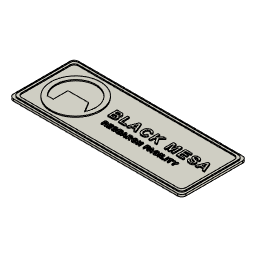
black_mesa_patch (Autodesk Fusion 360 design; units mm, degrees)
Autodesk Fusion 360 part; units mm, degrees
sketch "Sketch1" plane through (0, 0, 0) normal (0, 0, 1) x (1, 0, 0)
  line L0 (155.8764, -60.5348) -> (155.8764, -66.4765)
  line L1 (155.8764, -66.4765) -> (160.0294, -66.4765)
  spline S0 degree 3 poles (160.0294, -66.4765) (161.646, -66.4765) (162.6717, -66.4315) (163.1065, -66.3407) knots 0 0 0 0 1 1 1 1
  spline S1 degree 3 poles (163.1065, -66.3407) (163.7733, -66.219) (164.3166, -65.9235) (164.7355, -65.4534) knots 0 0 0 0 1 1 1 1
  spline S2 degree 3 poles (164.7355, -65.4534) (165.1553, -64.9833) (165.3643, -64.3545) (165.3643, -63.5661) knots 0 0 0 0 1 1 1 1
  spline S3 degree 3 poles (165.3643, -63.5661) (165.3643, -62.8993) (165.2029, -62.334) (164.8792, -61.8683) knots 0 0 0 0 1 1 1 1
  spline S4 degree 3 poles (164.8792, -61.8683) (164.5565, -61.4035) (164.089, -61.0657) (163.4778, -60.8532) knots 0 0 0 0 1 1 1 1
  spline S5 degree 3 poles (163.4778, -60.8532) (162.8658, -60.6407) (161.5402, -60.5348) (159.4985, -60.5348) knots 0 0 0 0 1 1 1 1
  line L2 (159.4985, -60.5348) -> (155.8764, -60.5348)
  line L3 (155.8764, -51.6977) -> (155.8764, -56.8368)
  line L4 (155.8764, -56.8368) -> (158.8168, -56.8368)
  spline S6 degree 3 poles (158.8168, -56.8368) (160.5648, -56.8368) (161.6513, -56.8112) (162.0755, -56.761) knots 0 0 0 0 1 1 1 1
  spline S7 degree 3 poles (162.0755, -56.761) (162.8437, -56.6701) (163.447, -56.4047) (163.8871, -55.9646) knots 0 0 0 0 1 1 1 1
  spline S8 degree 3 poles (163.8871, -55.9646) (164.3263, -55.5254) (164.5468, -54.9468) (164.5468, -54.2298) knots 0 0 0 0 1 1 1 1
  spline S9 degree 3 poles (164.5468, -54.2298) (164.5468, -53.5419) (164.3571, -52.9836) (163.9779, -52.555) knots 0 0 0 0 1 1 1 1
  spline S10 degree 3 poles (163.9779, -52.555) (163.5987, -52.1255) (163.036, -51.8644) (162.2881, -51.7736) knots 0 0 0 0 1 1 1 1
  spline S11 degree 3 poles (162.2881, -51.7736) (161.8436, -51.7233) (160.5648, -51.6977) (158.4534, -51.6977) knots 0 0 0 0 1 1 1 1
  line L5 (158.4534, -51.6977) -> (155.8764, -51.6977)
  line L6 (151.3899, -47.9997) -> (160.272, -47.9997)
  spline S12 degree 3 poles (160.272, -47.9997) (162.0306, -47.9997) (163.3411, -48.0729) (164.2054, -48.2193) knots 0 0 0 0 1 1 1 1
  spline S13 degree 3 poles (164.2054, -48.2193) (165.0689, -48.3666) (165.8423, -48.6718) (166.5241, -49.1366) knots 0 0 0 0 1 1 1 1
  spline S14 degree 3 poles (166.5241, -49.1366) (167.2067, -49.6014) (167.7747, -50.2205) (168.2298, -50.9931) knots 0 0 0 0 1 1 1 1
  spline S15 degree 3 poles (168.2298, -50.9931) (168.684, -51.7665) (168.9115, -52.6335) (168.9115, -53.593) knots 0 0 0 0 1 1 1 1
  spline S16 degree 3 poles (168.9115, -53.593) (168.9115, -54.6337) (168.631, -55.5889) (168.0701, -56.4576) knots 0 0 0 0 1 1 1 1
  spline S17 degree 3 poles (168.0701, -56.4576) (167.5092, -57.3263) (166.749, -57.9789) (165.7894, -58.4129) knots 0 0 0 0 1 1 1 1
  spline S18 degree 3 poles (165.7894, -58.4129) (167.1432, -58.8071) (168.1839, -59.4791) (168.9115, -60.429) knots 0 0 0 0 1 1 1 1
  spline S19 degree 3 poles (168.9115, -60.429) (169.6391, -61.3788) (170.0033, -62.4954) (170.0033, -63.7786) knots 0 0 0 0 1 1 1 1
  spline S20 degree 3 poles (170.0033, -63.7786) (170.0033, -64.7893) (169.7679, -65.7718) (169.2978, -66.727) knots 0 0 0 0 1 1 1 1
  spline S21 degree 3 poles (169.2978, -66.727) (168.8286, -67.6812) (168.1865, -68.4441) (167.3734, -69.0156) knots 0 0 0 0 1 1 1 1
  spline S22 degree 3 poles (167.3734, -69.0156) (166.5593, -69.5862) (165.5566, -69.9381) (164.3642, -70.0686) knots 0 0 0 0 1 1 1 1
  spline S23 degree 3 poles (164.3642, -70.0686) (163.6163, -70.1498) (161.8127, -70.2) (158.9535, -70.2203) knots 0 0 0 0 1 1 1 1
  line L7 (158.9535, -70.2203) -> (151.3899, -70.2203)
  line L8 (151.3899, -70.2203) -> (151.3899, -47.9997)
  line L9 (177.1731, -70.2203) -> (177.1731, -48.1814)
  line L10 (177.1731, -48.1814) -> (181.6596, -48.1814)
  line L11 (181.6596, -48.1814) -> (181.6596, -66.4765)
  line L12 (181.6596, -66.4765) -> (192.8153, -66.4765)
  line L13 (192.8153, -66.4765) -> (192.8153, -70.2203)
  line L14 (192.8153, -70.2203) -> (177.1731, -70.2203)
  line L15 (211.0496, -61.4293) -> (207.9875, -53.1831)
  line L16 (207.9875, -53.1831) -> (204.9871, -61.4293)
  line L17 (204.9871, -61.4293) -> (211.0496, -61.4293)
  line L18 (219.3107, -70.2205) -> (214.4301, -70.2205)
  line L19 (214.4301, -70.2205) -> (212.4898, -65.1731)
  line L20 (212.4898, -65.1731) -> (203.6077, -65.1731)
  line L21 (203.6077, -65.1731) -> (201.7733, -70.2205)
  line L22 (201.7733, -70.2205) -> (197.0143, -70.2205)
  line L23 (197.0143, -70.2205) -> (205.6688, -47.9999)
  line L24 (205.6688, -47.9999) -> (210.4128, -47.9999)
  line L25 (210.4128, -47.9999) -> (219.3107, -70.2205)
  line L26 (239.1675, -62.0507) -> (243.5182, -63.4301)
  spline S24 degree 3 poles (243.5182, -63.4301) (242.8505, -65.8545) (241.7411, -67.6563) (240.1906, -68.8329) knots 0 0 0 0 1 1 1 1
  spline S25 degree 3 poles (240.1906, -68.8329) (238.6384, -70.0111) (236.6716, -70.5994) (234.2869, -70.5994) knots 0 0 0 0 1 1 1 1
  spline S26 degree 3 poles (234.2869, -70.5994) (231.3359, -70.5994) (228.9105, -69.5913) (227.0117, -67.5752) knots 0 0 0 0 1 1 1 1
  spline S27 degree 3 poles (227.0117, -67.5752) (225.1111, -65.56) (224.1613, -62.8039) (224.1613, -59.307) knots 0 0 0 0 1 1 1 1
  spline S28 degree 3 poles (224.1613, -59.307) (224.1613, -55.609) (225.1164, -52.7365) (227.0258, -50.6904) knots 0 0 0 0 1 1 1 1
  spline S29 degree 3 poles (227.0258, -50.6904) (228.9361, -48.6443) (231.447, -47.6212) (234.5594, -47.6212) knots 0 0 0 0 1 1 1 1
  spline S30 degree 3 poles (234.5594, -47.6212) (237.2775, -47.6212) (239.485, -48.4238) (241.1828, -50.0307) knots 0 0 0 0 1 1 1 1
  spline S31 degree 3 poles (241.1828, -50.0307) (242.1935, -50.9805) (242.9511, -52.3449) (243.4564, -54.1238) knots 0 0 0 0 1 1 1 1
  line L27 (243.4564, -54.1238) -> (239.0158, -55.1839)
  spline S32 degree 3 poles (239.0158, -55.1839) (238.7521, -54.0321) (238.2045, -53.1228) (237.371, -52.456) knots 0 0 0 0 1 1 1 1
  spline S33 degree 3 poles (237.371, -52.456) (236.5376, -51.7893) (235.5242, -51.4559) (234.3327, -51.4559) knots 0 0 0 0 1 1 1 1
  spline S34 degree 3 poles (234.3327, -51.4559) (232.6844, -51.4559) (231.3491, -52.0468) (230.3234, -53.2295) knots 0 0 0 0 1 1 1 1
  spline S35 degree 3 poles (230.3234, -53.2295) (229.2977, -54.4113) (228.7853, -56.326) (228.7853, -58.9736) knots 0 0 0 0 1 1 1 1
  spline S36 degree 3 poles (228.7853, -58.9736) (228.7853, -61.7826) (229.2898, -63.7837) (230.3005, -64.9761) knots 0 0 0 0 1 1 1 1
  spline S37 degree 3 poles (230.3005, -64.9761) (231.3112, -66.1685) (232.6244, -66.7647) (234.241, -66.7647) knots 0 0 0 0 1 1 1 1
  spline S38 degree 3 poles (234.241, -66.7647) (235.4334, -66.7647) (236.4591, -66.3855) (237.3181, -65.6279) knots 0 0 0 0 1 1 1 1
  spline S39 degree 3 poles (237.3181, -65.6279) (238.1771, -64.8694) (238.7936, -63.6779) (239.1675, -62.0507) knots 0 0 0 0 1 1 1 1
  line L28 (250.6879, -70.2203) -> (250.6879, -47.9997)
  line L29 (250.6879, -47.9997) -> (255.1744, -47.9997)
  line L30 (255.1744, -47.9997) -> (255.1744, -57.8669)
  line L31 (255.1744, -57.8669) -> (264.2381, -47.9997)
  line L32 (264.2381, -47.9997) -> (270.2706, -47.9997)
  line L33 (270.2706, -47.9997) -> (261.9045, -56.6543)
  line L34 (261.9045, -56.6543) -> (270.7257, -70.2203)
  line L35 (270.7257, -70.2203) -> (264.9208, -70.2203)
  line L36 (264.9208, -70.2203) -> (258.8115, -59.7922)
  line L37 (258.8115, -59.7922) -> (255.1744, -63.5061)
  line L38 (255.1744, -63.5061) -> (255.1744, -70.2203)
  line L39 (255.1744, -70.2203) -> (250.6879, -70.2203)
  line L40 (288.1267, -70.2203) -> (288.1267, -47.9997)
  line L41 (288.1267, -47.9997) -> (294.8409, -47.9997)
  line L42 (294.8409, -47.9997) -> (298.8731, -63.1568)
  line L43 (298.8731, -63.1568) -> (302.8595, -47.9997)
  line L44 (302.8595, -47.9997) -> (309.5888, -47.9997)
  line L45 (309.5888, -47.9997) -> (309.5888, -70.2203)
  line L46 (309.5888, -70.2203) -> (305.4207, -70.2203)
  line L47 (305.4207, -70.2203) -> (305.4207, -52.7287)
  line L48 (305.4207, -52.7287) -> (301.0101, -70.2203)
  line L49 (301.0101, -70.2203) -> (296.6903, -70.2203)
  line L50 (296.6903, -70.2203) -> (292.2947, -52.7287)
  line L51 (292.2947, -52.7287) -> (292.2947, -70.2203)
  line L52 (292.2947, -70.2203) -> (288.1267, -70.2203)
  line L53 (317.3049, -70.2203) -> (317.3049, -47.9997)
  line L54 (317.3049, -47.9997) -> (333.7814, -47.9997)
  line L55 (333.7814, -47.9997) -> (333.7814, -51.7586)
  line L56 (333.7814, -51.7586) -> (321.7914, -51.7586)
  line L57 (321.7914, -51.7586) -> (321.7914, -56.6851)
  line L58 (321.7914, -56.6851) -> (332.9471, -56.6851)
  line L59 (332.9471, -56.6851) -> (332.9471, -60.429)
  line L60 (332.9471, -60.429) -> (321.7914, -60.429)
  line L61 (321.7914, -60.429) -> (321.7914, -66.4765)
  line L62 (321.7914, -66.4765) -> (334.2056, -66.4765)
  line L63 (334.2056, -66.4765) -> (334.2056, -70.2203)
  line L64 (334.2056, -70.2203) -> (317.3049, -70.2203)
  line L65 (340.1321, -62.9903) -> (344.4977, -62.5661)
  spline S40 degree 3 poles (344.4977, -62.5661) (344.7605, -64.031) (345.2941, -65.107) (346.0967, -65.794) knots 0 0 0 0 1 1 1 1
  spline S41 degree 3 poles (346.0967, -65.794) (346.9001, -66.4811) (347.9832, -66.825) (349.3475, -66.825) knots 0 0 0 0 1 1 1 1
  spline S42 degree 3 poles (349.3475, -66.825) (350.793, -66.825) (351.8814, -66.519) (352.6143, -65.9078) knots 0 0 0 0 1 1 1 1
  spline S43 degree 3 poles (352.6143, -65.9078) (353.3463, -65.2966) (353.7132, -64.5822) (353.7132, -63.7629) knots 0 0 0 0 1 1 1 1
  spline S44 degree 3 poles (353.7132, -63.7629) (353.7132, -63.2382) (353.5597, -62.791) (353.251, -62.4215) knots 0 0 0 0 1 1 1 1
  spline S45 degree 3 poles (353.251, -62.4215) (352.9423, -62.0528) (352.4044, -61.7327) (351.6371, -61.4593) knots 0 0 0 0 1 1 1 1
  spline S46 degree 3 poles (351.6371, -61.4593) (351.1105, -61.2776) (349.9137, -60.9539) (348.0449, -60.4891) knots 0 0 0 0 1 1 1 1
  spline S47 degree 3 poles (348.0449, -60.4891) (345.639, -59.8929) (343.9518, -59.1609) (342.9817, -58.2913) knots 0 0 0 0 1 1 1 1
  spline S48 degree 3 poles (342.9817, -58.2913) (341.6182, -57.069) (340.9355, -55.5785) (340.9355, -53.8208) knots 0 0 0 0 1 1 1 1
  spline S49 degree 3 poles (340.9355, -53.8208) (340.9355, -52.6883) (341.2557, -51.63) (341.8986, -50.6449) knots 0 0 0 0 1 1 1 1
  spline S50 degree 3 poles (341.8986, -50.6449) (342.5389, -49.6597) (343.4641, -48.9092) (344.6715, -48.3941) knots 0 0 0 0 1 1 1 1
  spline S51 degree 3 poles (344.6715, -48.3941) (345.8797, -47.8782) (347.3367, -47.6207) (349.0441, -47.6207) knots 0 0 0 0 1 1 1 1
  spline S52 degree 3 poles (349.0441, -47.6207) (351.8337, -47.6207) (353.9328, -48.2328) (355.343, -49.4551) knots 0 0 0 0 1 1 1 1
  spline S53 degree 3 poles (355.343, -49.4551) (356.7523, -50.6775) (357.4923, -52.31) (357.5637, -54.3508) knots 0 0 0 0 1 1 1 1
  line L66 (357.5637, -54.3508) -> (353.0773, -54.5475)
  spline S54 degree 3 poles (353.0773, -54.5475) (352.885, -53.4062) (352.4723, -52.5851) (351.8408, -52.0842) knots 0 0 0 0 1 1 1 1
  spline S55 degree 3 poles (351.8408, -52.0842) (351.2102, -51.5841) (350.2621, -51.3346) (348.9992, -51.3346) knots 0 0 0 0 1 1 1 1
  spline S56 degree 3 poles (348.9992, -51.3346) (347.6957, -51.3346) (346.6752, -51.6018) (345.9379, -52.138) knots 0 0 0 0 1 1 1 1
  spline S57 degree 3 poles (345.9379, -52.138) (345.4626, -52.4811) (345.2244, -52.9406) (345.2244, -53.5174) knots 0 0 0 0 1 1 1 1
  spline S58 degree 3 poles (345.2244, -53.5174) (345.2244, -54.0421) (345.4467, -54.4919) (345.8921, -54.8659) knots 0 0 0 0 1 1 1 1
  spline S59 degree 3 poles (345.8921, -54.8659) (346.4583, -55.3412) (347.8315, -55.836) (350.0152, -56.3519) knots 0 0 0 0 1 1 1 1
  spline S60 degree 3 poles (350.0152, -56.3519) (352.198, -56.867) (353.8119, -57.3997) (354.857, -57.9509) knots 0 0 0 0 1 1 1 1
  spline S61 degree 3 poles (354.857, -57.9509) (355.9039, -58.5012) (356.7224, -59.2544) (357.3124, -60.2087) knots 0 0 0 0 1 1 1 1
  spline S62 degree 3 poles (357.3124, -60.2087) (357.9042, -61.1638) (358.1996, -62.3439) (358.1996, -63.7479) knots 0 0 0 0 1 1 1 1
  spline S63 degree 3 poles (358.1996, -63.7479) (358.1996, -65.0214) (357.846, -66.2138) (357.1386, -67.3251) knots 0 0 0 0 1 1 1 1
  spline S64 degree 3 poles (357.1386, -67.3251) (356.4313, -68.4372) (355.4312, -69.2636) (354.1374, -69.8033) knots 0 0 0 0 1 1 1 1
  spline S65 degree 3 poles (354.1374, -69.8033) (352.8436, -70.344) (351.2323, -70.6147) (349.3017, -70.6147) knots 0 0 0 0 1 1 1 1
  spline S66 degree 3 poles (349.3017, -70.6147) (346.4936, -70.6147) (344.3363, -69.9656) (342.8308, -68.6665) knots 0 0 0 0 1 1 1 1
  spline S67 degree 3 poles (342.8308, -68.6665) (341.3254, -67.3683) (340.4249, -65.4756) (340.1321, -62.9903) knots 0 0 0 0 1 1 1 1
  line L67 (377.0102, -61.4293) -> (373.9481, -53.1831)
  line L68 (373.9481, -53.1831) -> (370.9477, -61.4293)
  line L69 (370.9477, -61.4293) -> (377.0102, -61.4293)
  line L70 (385.2713, -70.2205) -> (380.3907, -70.2205)
  line L71 (380.3907, -70.2205) -> (378.4504, -65.1731)
  line L72 (378.4504, -65.1731) -> (369.5683, -65.1731)
  line L73 (369.5683, -65.1731) -> (367.7339, -70.2205)
  line L74 (367.7339, -70.2205) -> (362.9749, -70.2205)
  line L75 (362.9749, -70.2205) -> (371.6294, -47.9999)
  line L76 (371.6294, -47.9999) -> (376.3734, -47.9999)
  line L77 (376.3734, -47.9999) -> (385.2713, -70.2205)
  line L78 (161.9462, -88.6895) -> (163.5663, -88.6895)
  spline S68 degree 3 poles (163.5663, -88.6895) (164.6176, -88.6895) (165.2737, -88.6445) (165.5357, -88.5563) knots 0 0 0 0 1 1 1 1
  spline S69 degree 3 poles (165.5357, -88.5563) (165.7967, -88.4672) (166.0013, -88.3138) (166.1495, -88.0968) knots 0 0 0 0 1 1 1 1
  spline S70 degree 3 poles (166.1495, -88.0968) (166.2977, -87.8799) (166.3718, -87.6082) (166.3718, -87.2828) knots 0 0 0 0 1 1 1 1
  spline S71 degree 3 poles (166.3718, -87.2828) (166.3718, -86.9177) (166.2739, -86.6231) (166.0798, -86.3982) knots 0 0 0 0 1 1 1 1
  spline S72 degree 3 poles (166.0798, -86.3982) (165.884, -86.1742) (165.6089, -86.0322) (165.2543, -85.9731) knots 0 0 0 0 1 1 1 1
  spline S73 degree 3 poles (165.2543, -85.9731) (165.0762, -85.9484) (164.5435, -85.9361) (163.6554, -85.9361) knots 0 0 0 0 1 1 1 1
  line L79 (163.6554, -85.9361) -> (161.9462, -85.9361)
  line L80 (161.9462, -85.9361) -> (161.9462, -88.6895)
  line L81 (159.7554, -94.9504) -> (159.7554, -84.1007)
  line L82 (159.7554, -84.1007) -> (164.3662, -84.1007)
  spline S74 degree 3 poles (164.3662, -84.1007) (165.526, -84.1007) (166.3682, -84.1977) (166.893, -84.3926) knots 0 0 0 0 1 1 1 1
  spline S75 degree 3 poles (166.893, -84.3926) (167.4186, -84.5884) (167.8393, -84.9342) (168.1551, -85.4333) knots 0 0 0 0 1 1 1 1
  spline S76 degree 3 poles (168.1551, -85.4333) (168.4708, -85.9308) (168.6287, -86.5014) (168.6287, -87.1426) knots 0 0 0 0 1 1 1 1
  spline S77 degree 3 poles (168.6287, -87.1426) (168.6287, -87.9566) (168.3896, -88.6286) (167.9108, -89.1587) knots 0 0 0 0 1 1 1 1
  spline S78 degree 3 poles (167.9108, -89.1587) (167.4327, -89.6896) (166.7166, -90.0239) (165.765, -90.1623) knots 0 0 0 0 1 1 1 1
  spline S79 degree 3 poles (165.765, -90.1623) (166.2386, -90.4375) (166.6293, -90.7418) (166.938, -91.0716) knots 0 0 0 0 1 1 1 1
  spline S80 degree 3 poles (166.938, -91.0716) (167.2458, -91.4023) (167.662, -91.9897) (168.185, -92.8329) knots 0 0 0 0 1 1 1 1
  line L83 (168.185, -92.8329) -> (169.5097, -94.9504)
  line L84 (169.5097, -94.9504) -> (166.8895, -94.9504)
  line L85 (166.8895, -94.9504) -> (165.3064, -92.5894)
  spline S81 degree 3 poles (165.3064, -92.5894) (164.7437, -91.7454) (164.3583, -91.2136) (164.151, -90.994) knots 0 0 0 0 1 1 1 1
  spline S82 degree 3 poles (164.151, -90.994) (163.9446, -90.7744) (163.725, -90.6245) (163.4922, -90.5433) knots 0 0 0 0 1 1 1 1
  spline S83 degree 3 poles (163.4922, -90.5433) (163.2611, -90.4622) (162.8934, -90.4207) (162.3898, -90.4207) knots 0 0 0 0 1 1 1 1
  line L86 (162.3898, -90.4207) -> (161.9462, -90.4207)
  line L87 (161.9462, -90.4207) -> (161.9462, -94.9504)
  line L88 (161.9462, -94.9504) -> (159.7554, -94.9504)
  line L89 (172.058, -94.9501) -> (172.058, -84.1004)
  line L90 (172.058, -84.1004) -> (180.1022, -84.1004)
  line L91 (180.1022, -84.1004) -> (180.1022, -85.9357)
  line L92 (180.1022, -85.9357) -> (174.2488, -85.9357)
  line L93 (174.2488, -85.9357) -> (174.2488, -88.3416)
  line L94 (174.2488, -88.3416) -> (179.6956, -88.3416)
  line L95 (179.6956, -88.3416) -> (179.6956, -90.169)
  line L96 (179.6956, -90.169) -> (174.2488, -90.169)
  line L97 (174.2488, -90.169) -> (174.2488, -93.1227)
  line L98 (174.2488, -93.1227) -> (180.3095, -93.1227)
  line L99 (180.3095, -93.1227) -> (180.3095, -94.9501)
  line L100 (180.3095, -94.9501) -> (172.058, -94.9501)
  line L101 (182.9763, -91.4197) -> (185.108, -91.2133)
  spline S84 degree 3 poles (185.108, -91.2133) (185.2358, -91.9277) (185.496, -92.4534) (185.8885, -92.7894) knots 0 0 0 0 1 1 1 1
  spline S85 degree 3 poles (185.8885, -92.7894) (186.2809, -93.1254) (186.8101, -93.2921) (187.476, -93.2921) knots 0 0 0 0 1 1 1 1
  spline S86 degree 3 poles (187.476, -93.2921) (188.1815, -93.2921) (188.7125, -93.143) (189.0705, -92.8441) knots 0 0 0 0 1 1 1 1
  spline S87 degree 3 poles (189.0705, -92.8441) (189.4277, -92.546) (189.6076, -92.1976) (189.6076, -91.7981) knots 0 0 0 0 1 1 1 1
  spline S88 degree 3 poles (189.6076, -91.7981) (189.6076, -91.5414) (189.5318, -91.3227) (189.3819, -91.1428) knots 0 0 0 0 1 1 1 1
  spline S89 degree 3 poles (189.3819, -91.1428) (189.2311, -90.962) (188.9682, -90.8059) (188.5934, -90.6718) knots 0 0 0 0 1 1 1 1
  spline S90 degree 3 poles (188.5934, -90.6718) (188.3368, -90.5836) (187.752, -90.4258) (186.8392, -90.1982) knots 0 0 0 0 1 1 1 1
  spline S91 degree 3 poles (186.8392, -90.1982) (185.6654, -89.9081) (184.8407, -89.55) (184.368, -89.1258) knots 0 0 0 0 1 1 1 1
  spline S92 degree 3 poles (184.368, -89.1258) (183.7013, -88.5287) (183.3688, -87.8002) (183.3688, -86.943) knots 0 0 0 0 1 1 1 1
  spline S93 degree 3 poles (183.3688, -86.943) (183.3688, -86.39) (183.5249, -85.8732) (183.8388, -85.3925) knots 0 0 0 0 1 1 1 1
  spline S94 degree 3 poles (183.8388, -85.3925) (184.1519, -84.911) (184.6035, -84.545) (185.1926, -84.2927) knots 0 0 0 0 1 1 1 1
  spline S95 degree 3 poles (185.1926, -84.2927) (185.7827, -84.0414) (186.4935, -83.9153) (187.3278, -83.9153) knots 0 0 0 0 1 1 1 1
  spline S96 degree 3 poles (187.3278, -83.9153) (188.6895, -83.9153) (189.7144, -84.2142) (190.4023, -84.8113) knots 0 0 0 0 1 1 1 1
  spline S97 degree 3 poles (190.4023, -84.8113) (191.0911, -85.4084) (191.4527, -86.2048) (191.4871, -87.2014) knots 0 0 0 0 1 1 1 1
  line L102 (191.4871, -87.2014) -> (189.2963, -87.2975)
  spline S98 degree 3 poles (189.2963, -87.2975) (189.2028, -86.7401) (189.0017, -86.3388) (188.6931, -86.0954) knots 0 0 0 0 1 1 1 1
  spline S99 degree 3 poles (188.6931, -86.0954) (188.3844, -85.8511) (187.9222, -85.7285) (187.3058, -85.7285) knots 0 0 0 0 1 1 1 1
  spline S100 degree 3 poles (187.3058, -85.7285) (186.669, -85.7285) (186.1707, -85.8591) (185.8109, -86.121) knots 0 0 0 0 1 1 1 1
  spline S101 degree 3 poles (185.8109, -86.121) (185.5789, -86.2894) (185.4625, -86.5135) (185.4625, -86.7948) knots 0 0 0 0 1 1 1 1
  spline S102 degree 3 poles (185.4625, -86.7948) (185.4625, -87.0514) (185.571, -87.2711) (185.7879, -87.4536) knots 0 0 0 0 1 1 1 1
  spline S103 degree 3 poles (185.7879, -87.4536) (186.0649, -87.6856) (186.736, -87.9272) (187.8014, -88.1786) knots 0 0 0 0 1 1 1 1
  spline S104 degree 3 poles (187.8014, -88.1786) (188.8668, -88.4299) (189.6553, -88.6901) (190.1659, -88.9591) knots 0 0 0 0 1 1 1 1
  spline S105 degree 3 poles (190.1659, -88.9591) (190.6766, -89.2281) (191.0761, -89.5959) (191.3645, -90.0624) knots 0 0 0 0 1 1 1 1
  spline S106 degree 3 poles (191.3645, -90.0624) (191.6538, -90.5281) (191.7975, -91.1049) (191.7975, -91.7901) knots 0 0 0 0 1 1 1 1
  spline S107 degree 3 poles (191.7975, -91.7901) (191.7975, -92.4119) (191.6255, -92.994) (191.2798, -93.5364) knots 0 0 0 0 1 1 1 1
  spline S108 degree 3 poles (191.2798, -93.5364) (190.9341, -94.0797) (190.4455, -94.4827) (189.814, -94.7464) knots 0 0 0 0 1 1 1 1
  spline S109 degree 3 poles (189.814, -94.7464) (189.1825, -95.0101) (188.3959, -95.1424) (187.4539, -95.1424) knots 0 0 0 0 1 1 1 1
  spline S110 degree 3 poles (187.4539, -95.1424) (186.0816, -95.1424) (185.0286, -94.8249) (184.2939, -94.1917) knots 0 0 0 0 1 1 1 1
  spline S111 degree 3 poles (184.2939, -94.1917) (183.5584, -93.5576) (183.1192, -92.6333) (182.9763, -91.4197) knots 0 0 0 0 1 1 1 1
  line L103 (195.0049, -94.9501) -> (195.0049, -84.1004)
  line L104 (195.0049, -84.1004) -> (203.0491, -84.1004)
  line L105 (203.0491, -84.1004) -> (203.0491, -85.9357)
  line L106 (203.0491, -85.9357) -> (197.1956, -85.9357)
  line L107 (197.1956, -85.9357) -> (197.1956, -88.3416)
  line L108 (197.1956, -88.3416) -> (202.6425, -88.3416)
  line L109 (202.6425, -88.3416) -> (202.6425, -90.169)
  line L110 (202.6425, -90.169) -> (197.1956, -90.169)
  line L111 (197.1956, -90.169) -> (197.1956, -93.1227)
  line L112 (197.1956, -93.1227) -> (203.2564, -93.1227)
  line L113 (203.2564, -93.1227) -> (203.2564, -94.9501)
  line L114 (203.2564, -94.9501) -> (195.0049, -94.9501)
  line L115 (212.2286, -90.6575) -> (210.7337, -86.6323)
  line L116 (210.7337, -86.6323) -> (209.2688, -90.6575)
  line L117 (209.2688, -90.6575) -> (212.2286, -90.6575)
  line L118 (216.2618, -94.9499) -> (213.8788, -94.9499)
  line L119 (213.8788, -94.9499) -> (212.9315, -92.4857)
  line L120 (212.9315, -92.4857) -> (208.595, -92.4857)
  line L121 (208.595, -92.4857) -> (207.699, -94.9499)
  line L122 (207.699, -94.9499) -> (205.375, -94.9499)
  line L123 (205.375, -94.9499) -> (209.6013, -84.1002)
  line L124 (209.6013, -84.1002) -> (211.9173, -84.1002)
  line L125 (211.9173, -84.1002) -> (216.2618, -94.9499)
  line L126 (220.9852, -88.6895) -> (222.6062, -88.6895)
  spline S112 degree 3 poles (222.6062, -88.6895) (223.6566, -88.6895) (224.3128, -88.6445) (224.5747, -88.5563) knots 0 0 0 0 1 1 1 1
  spline S113 degree 3 poles (224.5747, -88.5563) (224.8358, -88.4672) (225.0413, -88.3138) (225.1894, -88.0968) knots 0 0 0 0 1 1 1 1
  spline S114 degree 3 poles (225.1894, -88.0968) (225.3376, -87.8799) (225.4117, -87.6082) (225.4117, -87.2828) knots 0 0 0 0 1 1 1 1
  spline S115 degree 3 poles (225.4117, -87.2828) (225.4117, -86.9177) (225.3138, -86.6231) (225.1189, -86.3982) knots 0 0 0 0 1 1 1 1
  spline S116 degree 3 poles (225.1189, -86.3982) (224.924, -86.1742) (224.6488, -86.0322) (224.2934, -85.9731) knots 0 0 0 0 1 1 1 1
  spline S117 degree 3 poles (224.2934, -85.9731) (224.1161, -85.9484) (223.5825, -85.9361) (222.6944, -85.9361) knots 0 0 0 0 1 1 1 1
  line L127 (222.6944, -85.9361) -> (220.9852, -85.9361)
  line L128 (220.9852, -85.9361) -> (220.9852, -88.6895)
  line L129 (218.7953, -94.9504) -> (218.7953, -84.1007)
  line L130 (218.7953, -84.1007) -> (223.4053, -84.1007)
  spline S118 degree 3 poles (223.4053, -84.1007) (224.565, -84.1007) (225.4081, -84.1977) (225.9329, -84.3926) knots 0 0 0 0 1 1 1 1
  spline S119 degree 3 poles (225.9329, -84.3926) (226.4585, -84.5884) (226.8792, -84.9342) (227.195, -85.4333) knots 0 0 0 0 1 1 1 1
  spline S120 degree 3 poles (227.195, -85.4333) (227.5098, -85.9308) (227.6686, -86.5014) (227.6686, -87.1426) knots 0 0 0 0 1 1 1 1
  spline S121 degree 3 poles (227.6686, -87.1426) (227.6686, -87.9566) (227.4296, -88.6286) (226.9507, -89.1587) knots 0 0 0 0 1 1 1 1
  spline S122 degree 3 poles (226.9507, -89.1587) (226.4718, -89.6896) (225.7565, -90.0239) (224.804, -90.1623) knots 0 0 0 0 1 1 1 1
  spline S123 degree 3 poles (224.804, -90.1623) (225.2776, -90.4375) (225.6692, -90.7418) (225.977, -91.0716) knots 0 0 0 0 1 1 1 1
  spline S124 degree 3 poles (225.977, -91.0716) (226.2857, -91.4023) (226.7011, -91.9897) (227.2241, -92.8329) knots 0 0 0 0 1 1 1 1
  line L131 (227.2241, -92.8329) -> (228.5488, -94.9504)
  line L132 (228.5488, -94.9504) -> (225.9285, -94.9504)
  line L133 (225.9285, -94.9504) -> (224.3454, -92.5894)
  spline S125 degree 3 poles (224.3454, -92.5894) (223.7827, -91.7454) (223.3982, -91.2136) (223.1909, -90.994) knots 0 0 0 0 1 1 1 1
  spline S126 degree 3 poles (223.1909, -90.994) (222.9837, -90.7744) (222.7641, -90.6245) (222.5321, -90.5433) knots 0 0 0 0 1 1 1 1
  spline S127 degree 3 poles (222.5321, -90.5433) (222.3002, -90.4622) (221.9324, -90.4207) (221.4297, -90.4207) knots 0 0 0 0 1 1 1 1
  line L134 (221.4297, -90.4207) -> (220.9852, -90.4207)
  line L135 (220.9852, -90.4207) -> (220.9852, -94.9504)
  line L136 (220.9852, -94.9504) -> (218.7953, -94.9504)
  line L137 (238.0393, -90.9615) -> (240.163, -91.6344)
  spline S128 degree 3 poles (240.163, -91.6344) (239.8376, -92.818) (239.2969, -93.6981) (238.5384, -94.2732) knots 0 0 0 0 1 1 1 1
  spline S129 degree 3 poles (238.5384, -94.2732) (237.7817, -94.8473) (236.8204, -95.1348) (235.6563, -95.1348) knots 0 0 0 0 1 1 1 1
  spline S130 degree 3 poles (235.6563, -95.1348) (234.216, -95.1348) (233.0316, -94.6427) (232.1047, -93.6593) knots 0 0 0 0 1 1 1 1
  spline S131 degree 3 poles (232.1047, -93.6593) (231.1769, -92.6742) (230.7121, -91.3283) (230.7121, -89.6209) knots 0 0 0 0 1 1 1 1
  spline S132 degree 3 poles (230.7121, -89.6209) (230.7121, -87.8164) (231.1795, -86.4133) (232.1117, -85.414) knots 0 0 0 0 1 1 1 1
  spline S133 degree 3 poles (232.1117, -85.414) (233.0439, -84.4148) (234.2707, -83.9156) (235.7894, -83.9156) knots 0 0 0 0 1 1 1 1
  spline S134 degree 3 poles (235.7894, -83.9156) (237.1168, -83.9156) (238.1954, -84.3081) (239.0235, -85.0921) knots 0 0 0 0 1 1 1 1
  spline S135 degree 3 poles (239.0235, -85.0921) (239.5174, -85.556) (239.8878, -86.2219) (240.1339, -87.0906) knots 0 0 0 0 1 1 1 1
  line L138 (240.1339, -87.0906) -> (237.9652, -87.6083)
  spline S136 degree 3 poles (237.9652, -87.6083) (237.8373, -87.0465) (237.5701, -86.602) (237.1626, -86.2757) knots 0 0 0 0 1 1 1 1
  spline S137 degree 3 poles (237.1626, -86.2757) (236.7552, -85.9503) (236.2604, -85.788) (235.6783, -85.788) knots 0 0 0 0 1 1 1 1
  spline S138 degree 3 poles (235.6783, -85.788) (234.874, -85.788) (234.2222, -86.0764) (233.7213, -86.654) knots 0 0 0 0 1 1 1 1
  spline S139 degree 3 poles (233.7213, -86.654) (233.2203, -87.2317) (232.9699, -88.1657) (232.9699, -89.4586) knots 0 0 0 0 1 1 1 1
  spline S140 degree 3 poles (232.9699, -89.4586) (232.9699, -90.8309) (233.2168, -91.8072) (233.7107, -92.3893) knots 0 0 0 0 1 1 1 1
  spline S141 degree 3 poles (233.7107, -92.3893) (234.2028, -92.9714) (234.8449, -93.2625) (235.6342, -93.2625) knots 0 0 0 0 1 1 1 1
  spline S142 degree 3 poles (235.6342, -93.2625) (236.2172, -93.2625) (236.7172, -93.0772) (237.137, -92.7068) knots 0 0 0 0 1 1 1 1
  spline S143 degree 3 poles (237.137, -92.7068) (237.556, -92.3382) (237.8567, -91.7552) (238.0393, -90.9615) knots 0 0 0 0 1 1 1 1
  line L139 (243.4145, -94.9501) -> (243.4145, -84.1004)
  line L140 (243.4145, -84.1004) -> (245.6044, -84.1004)
  line L141 (245.6044, -84.1004) -> (245.6044, -88.3707)
  line L142 (245.6044, -88.3707) -> (249.8977, -88.3707)
  line L143 (249.8977, -88.3707) -> (249.8977, -84.1004)
  line L144 (249.8977, -84.1004) -> (252.0885, -84.1004)
  line L145 (252.0885, -84.1004) -> (252.0885, -94.9501)
  line L146 (252.0885, -94.9501) -> (249.8977, -94.9501)
  line L147 (249.8977, -94.9501) -> (249.8977, -90.2061)
  line L148 (249.8977, -90.2061) -> (245.6044, -90.2061)
  line L149 (245.6044, -90.2061) -> (245.6044, -94.9501)
  line L150 (245.6044, -94.9501) -> (243.4145, -94.9501)
  line L151 (261.3074, -94.9501) -> (261.3074, -84.1004)
  line L152 (261.3074, -84.1004) -> (268.7449, -84.1004)
  line L153 (268.7449, -84.1004) -> (268.7449, -85.9357)
  line L154 (268.7449, -85.9357) -> (263.4973, -85.9357)
  line L155 (263.4973, -85.9357) -> (263.4973, -88.5039)
  line L156 (263.4973, -88.5039) -> (268.027, -88.5039)
  line L157 (268.027, -88.5039) -> (268.027, -90.3392)
  line L158 (268.027, -90.3392) -> (263.4973, -90.3392)
  line L159 (263.4973, -90.3392) -> (263.4973, -94.9501)
  line L160 (263.4973, -94.9501) -> (261.3074, -94.9501)
  line L161 (276.8285, -90.6575) -> (275.3336, -86.6323)
  line L162 (275.3336, -86.6323) -> (273.8687, -90.6575)
  line L163 (273.8687, -90.6575) -> (276.8285, -90.6575)
  line L164 (280.8616, -94.9499) -> (278.4786, -94.9499)
  line L165 (278.4786, -94.9499) -> (277.5314, -92.4857)
  line L166 (277.5314, -92.4857) -> (273.1949, -92.4857)
  line L167 (273.1949, -92.4857) -> (272.2988, -94.9499)
  line L168 (272.2988, -94.9499) -> (269.9749, -94.9499)
  line L169 (269.9749, -94.9499) -> (274.2012, -84.1002)
  line L170 (274.2012, -84.1002) -> (276.5172, -84.1002)
  line L171 (276.5172, -84.1002) -> (280.8616, -94.9499)
  line L172 (290.329, -90.9615) -> (292.4527, -91.6344)
  spline S144 degree 3 poles (292.4527, -91.6344) (292.1272, -92.818) (291.5866, -93.6981) (290.8281, -94.2732) knots 0 0 0 0 1 1 1 1
  spline S145 degree 3 poles (290.8281, -94.2732) (290.0714, -94.8473) (289.1101, -95.1348) (287.9459, -95.1348) knots 0 0 0 0 1 1 1 1
  spline S146 degree 3 poles (287.9459, -95.1348) (286.5057, -95.1348) (285.3213, -94.6427) (284.3944, -93.6593) knots 0 0 0 0 1 1 1 1
  spline S147 degree 3 poles (284.3944, -93.6593) (283.4666, -92.6742) (283.0018, -91.3283) (283.0018, -89.6209) knots 0 0 0 0 1 1 1 1
  spline S148 degree 3 poles (283.0018, -89.6209) (283.0018, -87.8164) (283.4692, -86.4133) (284.4014, -85.414) knots 0 0 0 0 1 1 1 1
  spline S149 degree 3 poles (284.4014, -85.414) (285.3336, -84.4148) (286.5604, -83.9156) (288.0791, -83.9156) knots 0 0 0 0 1 1 1 1
  spline S150 degree 3 poles (288.0791, -83.9156) (289.4064, -83.9156) (290.4851, -84.3081) (291.3132, -85.0921) knots 0 0 0 0 1 1 1 1
  spline S151 degree 3 poles (291.3132, -85.0921) (291.8071, -85.556) (292.1775, -86.2219) (292.4236, -87.0906) knots 0 0 0 0 1 1 1 1
  line L173 (292.4236, -87.0906) -> (290.2549, -87.6083)
  spline S152 degree 3 poles (290.2549, -87.6083) (290.127, -87.0465) (289.8598, -86.602) (289.4523, -86.2757) knots 0 0 0 0 1 1 1 1
  spline S153 degree 3 poles (289.4523, -86.2757) (289.0448, -85.9503) (288.5501, -85.788) (287.968, -85.788) knots 0 0 0 0 1 1 1 1
  spline S154 degree 3 poles (287.968, -85.788) (287.1637, -85.788) (286.5119, -86.0764) (286.011, -86.654) knots 0 0 0 0 1 1 1 1
  spline S155 degree 3 poles (286.011, -86.654) (285.51, -87.2317) (285.2595, -88.1657) (285.2595, -89.4586) knots 0 0 0 0 1 1 1 1
  spline S156 degree 3 poles (285.2595, -89.4586) (285.2595, -90.8309) (285.5065, -91.8072) (286.0004, -92.3893) knots 0 0 0 0 1 1 1 1
  spline S157 degree 3 poles (286.0004, -92.3893) (286.4925, -92.9714) (287.1346, -93.2625) (287.9239, -93.2625) knots 0 0 0 0 1 1 1 1
  spline S158 degree 3 poles (287.9239, -93.2625) (288.5069, -93.2625) (289.0069, -93.0772) (289.4267, -92.7068) knots 0 0 0 0 1 1 1 1
  spline S159 degree 3 poles (289.4267, -92.7068) (289.8457, -92.3382) (290.1464, -91.7552) (290.329, -90.9615) knots 0 0 0 0 1 1 1 1
  line L174 (295.6313, -84.1005) -> (297.8212, -84.1005)
  line L175 (297.8212, -84.1005) -> (297.8212, -94.9501)
  line L176 (297.8212, -94.9501) -> (295.6313, -94.9501)
  line L177 (295.6313, -94.9501) -> (295.6313, -84.1005)
  line L178 (301.3317, -94.9501) -> (301.3317, -84.1894)
  line L179 (301.3317, -84.1894) -> (303.5225, -84.1894)
  line L180 (303.5225, -84.1894) -> (303.5225, -93.1227)
  line L181 (303.5225, -93.1227) -> (308.9694, -93.1227)
  line L182 (308.9694, -93.1227) -> (308.9694, -94.9501)
  line L183 (308.9694, -94.9501) -> (301.3317, -94.9501)
  line L184 (311.8282, -84.1005) -> (314.0181, -84.1005)
  line L185 (314.0181, -84.1005) -> (314.0181, -94.9501)
  line L186 (314.0181, -94.9501) -> (311.8282, -94.9501)
  line L187 (311.8282, -94.9501) -> (311.8282, -84.1005)
  line L188 (319.912, -94.9501) -> (319.912, -85.9357)
  line L189 (319.912, -85.9357) -> (316.6929, -85.9357)
  line L190 (316.6929, -85.9357) -> (316.6929, -84.1004)
  line L191 (316.6929, -84.1004) -> (325.3148, -84.1004)
  line L192 (325.3148, -84.1004) -> (325.3148, -85.9357)
  line L193 (325.3148, -85.9357) -> (322.1019, -85.9357)
  line L194 (322.1019, -85.9357) -> (322.1019, -94.9501)
  line L195 (322.1019, -94.9501) -> (319.912, -94.9501)
  line L196 (330.9414, -94.9501) -> (330.9414, -90.3833)
  line L197 (330.9414, -90.3833) -> (326.9665, -84.1004)
  line L198 (326.9665, -84.1004) -> (329.5347, -84.1004)
  line L199 (329.5347, -84.1004) -> (332.088, -88.3928)
  line L200 (332.088, -88.3928) -> (334.59, -84.1004)
  line L201 (334.59, -84.1004) -> (337.1133, -84.1004)
  line L202 (337.1133, -84.1004) -> (333.1243, -90.3983)
  line L203 (333.1243, -90.3983) -> (333.1243, -94.9501)
  line L204 (333.1243, -94.9501) -> (330.9414, -94.9501)
  line L205 (101.3586, -66.9474) -> (51.6311, -66.9474)
  line L206 (51.6311, -66.9474) -> (51.6311, -102.5118)
  line L207 (51.6311, -102.5118) -> (37.191, -102.5118)
  spline S160 degree 3 poles (37.191, -102.5118) (28.7437, -93.7682) (23.5438, -81.8655) (23.5438, -68.7492) knots 0 0 0 0 1 1 1 1
  spline S161 degree 3 poles (23.5438, -68.7492) (23.5438, -41.9143) (45.2978, -20.1594) (72.1345, -20.1594) knots 0 0 0 0 1 1 1 1
  spline S162 degree 3 poles (72.1345, -20.1594) (98.9703, -20.1594) (120.7244, -41.9143) (120.7244, -68.7492) knots 0 0 0 0 1 1 1 1
  spline S163 degree 3 poles (120.7244, -68.7492) (120.7244, -76.6303) (118.8458, -84.0766) (115.5138, -90.6603) knots 0 0 0 0 1 1 1 1
  line L208 (115.5138, -90.6603) -> (101.3586, -66.9474)
  spline S164 degree 3 poles (72.1345, -9.1166) (39.2, -9.1166) (12.5001, -35.8148) (12.5001, -68.7492) knots 0 0 0 0 1 1 1 1
  spline S165 degree 3 poles (12.5001, -68.7492) (12.5001, -101.6855) (39.2001, -128.3828) (72.1345, -128.3828) knots 0 0 0 0 1 1 1 1
  spline S166 degree 3 poles (72.1345, -128.3828) (105.0689, -128.3828) (131.7672, -101.6855) (131.7672, -68.7492) knots 0 0 0 0 1 1 1 1
  spline S167 degree 3 poles (131.7672, -68.7492) (131.7672, -35.8148) (105.0689, -9.1166) (72.1345, -9.1166) knots 0 0 0 0 1 1 1 1
  line L209 (10, 0) -> (387.7713, 0)
  line L210 (397.7713, -10) -> (397.7713, -127.4998)
  line L211 (387.7713, -137.4998) -> (10, -137.4998)
  line L212 (0, -127.4998) -> (0, -10)
  line L213 (0, 10) -> (397.7713, 10)
  line L214 (407.7713, 0) -> (407.7713, -137.4998)
  line L215 (397.7713, -147.4998) -> (0, -147.4998)
  line L216 (-10, -137.4998) -> (-10, 0)
  arc A0 (10, 0) -> (0, -10) centre (10, -10) ccw
  arc A1 (0, -127.4998) -> (10, -137.4998) centre (10, -127.4998) ccw
  arc A2 (387.7713, -137.4998) -> (397.7713, -127.4998) centre (387.7713, -127.4998) ccw
  arc A3 (397.7713, -10) -> (387.7713, 0) centre (387.7713, -10) ccw
  arc A4 (407.7713, 0) -> (397.7713, 10) centre (397.7713, 0) ccw
  arc A5 (0, 10) -> (-10, 0) centre (0, 0) ccw
  arc A6 (-10, -137.4998) -> (0, -147.4998) centre (0, -137.4998) ccw
  arc A7 (397.7713, -147.4998) -> (407.7713, -137.4998) centre (397.7713, -137.4998) ccw
  line L217 (5, 5) -> (392.7713, 5)
  line L218 (402.7713, -5) -> (402.7713, -132.4998)
  line L219 (392.7713, -142.4998) -> (5, -142.4998)
  line L220 (-5, -132.4998) -> (-5, -5)
  arc A8 (5, 5) -> (-5, -5) centre (5, -5) ccw
  arc A9 (402.7713, -5) -> (392.7713, 5) centre (392.7713, -5) ccw
  arc A10 (392.7713, -142.4998) -> (402.7713, -132.4998) centre (392.7713, -132.4998) ccw
  arc A11 (-5, -132.4998) -> (5, -142.4998) centre (5, -132.4998) ccw
  dimension "d1" = 9.1166
  dimension "d2" = 12.5001
  dimension "d3" = 12.5
  dimension "d4" = 9.117
  dimension "d5" = 10
  dimension "d6" = 10
  dimension "d7" = 10
  dimension "d8" = 10
  dimension "d9" = 10
  dimension "d10" = 10
  dimension "d11" = 10
  dimension "d12" = 10
  dimension "d13" = 10
  dimension "d14" = 10
  dimension "d15" = 10
  dimension "d16" = 10
  dimension "d17" = 10
  dimension "d18" = 10
  dimension "d19" = 10
  dimension "d20" = 10
  dimension "d21" = 5
  dimension "d22" = 5
  dimension "d23" = 5
  dimension "d24" = 5
  constraint horizontal L209
  constraint vertical L210
  constraint horizontal L211
  constraint vertical L212
  constraint horizontal L213
  constraint vertical L214
  constraint horizontal L215
  constraint vertical L216
  constraint tangent L209 A0
  constraint tangent L212 A0
  constraint tangent L211 A1
  constraint tangent L212 A1
  constraint tangent L210 A2
  constraint tangent L211 A2
  constraint tangent L209 A3
  constraint tangent L210 A3
  constraint tangent L213 A4
  constraint tangent L214 A4
  constraint tangent L213 A5
  constraint tangent L216 A5
  constraint tangent L215 A6
  constraint tangent L216 A6
  constraint tangent L214 A7
  constraint tangent L215 A7
  constraint horizontal L217
  constraint vertical L218
  constraint horizontal L219
  constraint vertical L220
  constraint tangent L217 A8
  constraint tangent L220 A8
  constraint tangent L217 A9
  constraint tangent L218 A9
  constraint tangent L218 A10
  constraint tangent L219 A10
  constraint tangent L219 A11
  constraint tangent L220 A11
  measures "d1" distance of S164.start L209
  measures "d2" distance of S164.end L212
  measures "d3" distance of L70.start L210
  measures "d4" distance of S165.end L211
  measures "d5" radius of A0
  measures "d6" radius of A1
  measures "d7" radius of A2
  measures "d8" radius of A3
  measures "d9" radius of A4
  measures "d10" radius of A5
  measures "d11" radius of A6
  measures "d12" radius of A7
  measures "d13" distance of L209 L213
  measures "d14" distance of L211 L215
  measures "d15" distance of L212 L216
  measures "d16" distance of L210 L214
  measures "d17" radius of A8
  measures "d18" radius of A9
  measures "d19" radius of A10
  measures "d20" radius of A11
  measures "d21" distance of L212 L220
  measures "d22" distance of L209 L217
  measures "d23" distance of L211 L219
  measures "d24" distance of L214 L218
extrude "Extrude1" add sketch "Sketch1" against normal blind 5 contours L0 L1 S0 S1 S2 S3 S4 S5 L2 | L3 L4 S6 S7 S8 S9 S10 S11 L5 | L6 S12 S13 S14 S15 S16 S17 S18 S19 S20 S21 S22 S23 L7 L8 | L9 L10 L11 L12 L13 L14 | L15 L16 L17 | L18 L19 L20 L21 L22 L23 L24 L25 | L26 S24 S25 S26 S27 S28 S29 S30 S31 L27 S32 S33 S34 S35 S36 S37 S38 S39 | L28 L29 L30 L31 L32 L33 L34 L35 L36 L37 L38 L39 | L40 L41 L42 L43 L44 L45 L46 L47 L48 L49 L50 L51 L52 | L53 L54 L55 L56 L57 L58 L59 L60 L61 L62 L63 L64 | L65 S40 S41 S42 S43 S44 S45 S46 S47 S48 S49 S50 S51 S52 S53 L66 S54 S55 S56 S57 S58 S59 S60 S61 S62 S63 S64 S65 S66 S67 | L67 L68 L69 | L70 L71 L72 L73 L74 L75 L76 L77 | L78 S68 S69 S70 S71 S72 S73 L79 L80 | L81 L82 S74 S75 S76 S77 S78 S79 S80 L83 L84 L85 S81 S82 S83 L86 L87 L88 | L89 L90 L91 L92 L93 L94 L95 L96 L97 L98 L99 L100 | L101 S84 S85 S86 S87 S88 S89 S90 S91 S92 S93 S94 S95 S96 S97 L102 S98 S99 S100 S101 S102 S103 S104 S105 S106 S107 S108 S109 S110 S111 | L103 L104 L105 L106 L107 L108 L109 L110 L111 L112 L113 L114 | L115 L116 L117 | L118 L119 L120 L121 L122 L123 L124 L125 | L126 S112 S113 S114 S115 S116 S117 L127 L128 | L129 L130 S118 S119 S120 S121 S122 S123 S124 L131 L132 L133 S125 S126 S127 L134 L135 L136 | L137 S128 S129 S130 S131 S132 S133 S134 S135 L138 S136 S137 S138 S139 S140 S141 S142 S143 | L139 L140 L141 L142 L143 L144 L145 L146 L147 L148 L149 L150 | L151 L152 L153 L154 L155 L156 L157 L158 L159 L160 | L161 L162 L163 | L164 L165 L166 L167 L168 L169 L170 L171 | L172 S144 S145 S146 S147 S148 S149 S150 S151 L173 S152 S153 S154 S155 S156 S157 S158 S159 | L174 L175 L176 L177 | L178 L179 L180 L181 L182 L183 | L184 L185 L186 L187 | L188 L189 L190 L191 L192 L193 L194 L195 | L196 L197 L198 L199 L200 L201 L202 L203 L204 | L205 L206 L207 S160 S161 S162 S163 L208 | S164 S165 S166 S167 | L209 L210 L211 L212 A0 A1 A2 A3 | L213 L214 L215 L216 A4 A5 A6 A7 | L217 L218 L219 L220 A8 A9 A10 A11
extrude "Extrude2" add sketch "Sketch1" along normal blind 2.5 contours L6 S12 S13 S14 S15 S16 S17 S18 S19 S20 S21 S22 S23 L7 L8 | L9 L10 L11 L12 L13 L14 | L18 L19 L20 L21 L22 L23 L24 L25 | L26 S24 S25 S26 S27 S28 S29 S30 S31 L27 S32 S33 S34 S35 S36 S37 S38 S39 | L28 L29 L30 L31 L32 L33 L34 L35 L36 L37 L38 L39 | L40 L41 L42 L43 L44 L45 L46 L47 L48 L49 L50 L51 L52 | L53 L54 L55 L56 L57 L58 L59 L60 L61 L62 L63 L64 | L65 S40 S41 S42 S43 S44 S45 S46 S47 S48 S49 S50 S51 S52 S53 L66 S54 S55 S56 S57 S58 S59 S60 S61 S62 S63 S64 S65 S66 S67 | L70 L71 L72 L73 L74 L75 L76 L77 | L81 L82 S74 S75 S76 S77 S78 S79 S80 L83 L84 L85 S81 S82 S83 L86 L87 L88 | L89 L90 L91 L92 L93 L94 L95 L96 L97 L98 L99 L100 | L101 S84 S85 S86 S87 S88 S89 S90 S91 S92 S93 S94 S95 S96 S97 L102 S98 S99 S100 S101 S102 S103 S104 S105 S106 S107 S108 S109 S110 S111 | L103 L104 L105 L106 L107 L108 L109 L110 L111 L112 L113 L114 | L118 L119 L120 L121 L122 L123 L124 L125 | L129 L130 S118 S119 S120 S121 S122 S123 S124 L131 L132 L133 S125 S126 S127 L134 L135 L136 | L137 S128 S129 S130 S131 S132 S133 S134 S135 L138 S136 S137 S138 S139 S140 S141 S142 S143 | L139 L140 L141 L142 L143 L144 L145 L146 L147 L148 L149 L150 | L151 L152 L153 L154 L155 L156 L157 L158 L159 L160 | L164 L165 L166 L167 L168 L169 L170 L171 | L172 S144 S145 S146 S147 S148 S149 S150 S151 L173 S152 S153 S154 S155 S156 S157 S158 S159 | L174 L175 L176 L177 | L178 L179 L180 L181 L182 L183 | L184 L185 L186 L187 | L188 L189 L190 L191 L192 L193 L194 L195 | L196 L197 L198 L199 L200 L201 L202 L203 L204 | S164 S165 S166 S167 | L217 L218 L219 L220 A8 A9 A10 A11
scale "Scale1" factor 0.45 about (397.7713, -147.4998, 0) bodies 1
